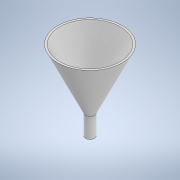
# Autodesk Inventor part: funnellForLogSplitter
Saved by Autodesk Inventor 2020.2 (Build 242310000, 310)
## iProperties
Created: 2019-12-25
Part Number: funnellForLogSplitter
Material: Generic
Document SubType Name: Modeling
Designer: robst
Density: 1 g/cm^3
Appearance: Default
Author: robst
Autodesk Inventor part; units mm, degrees
ref_plane "YZ Plane" through (0, 0, 0) normal (1, 0, 0) x (0, 1, 0)
ref_plane "XZ Plane" through (0, 0, 0) normal (0, 1, 0) x (-1, 0, 0)
ref_plane "XY Plane" through (0, 0, 0) normal (0, 0, 1) x (1, 0, 0)
sketch "Sketch1" plane through (0, 0, 0) normal (0, 0, 1) x (1, 0, 0)
  line L0 (5.715, 0) -> (5.715, 25.4)
  line L1 (5.715, 25.4) -> (41.275, 101.6)
  line L2 (41.275, 101.6) -> (38.735, 101.6)
  line L3 (38.735, 101.6) -> (3.175, 25.4)
  line L4 (3.175, 25.4) -> (3.175, 0)
  line L5 (3.175, 0) -> (5.715, 0)
  line L6 (0, 0) -> (5.715, 0) construction
  line L7 (0, 0) -> (0, 101.6) construction
  line L8 (5.715, 25.4) -> (71.0866, 25.4) construction
  dimension "d0" = 2.54
  dimension "d1" = 5.715
  dimension "d2" = 25.4
  dimension "d3" = 101.6
  dimension "d4" = 41.275
  dimension "d7" = 76.2
  constraints: 18 end point, 3 parallel, 3 perpendicular, 2 vertical, 1 collinear, 1 horizontal, 1 point on line
  measures "d0" distance between parallel lines of L4 L0
  measures "d1" distance of L0.start L6.start
  measures "d2" distance of L0.start L0.end
  measures "d3" distance of L6.start L7.end
  measures "d4" distance from line of L7 L1.end
  measures "d7" distance from line of L1.end L8
revolve "Revolution1" add sketch "Sketch1" angle 360 about axis through (0, 0, 0) along (0, 1, 0)
body "Solid1"
